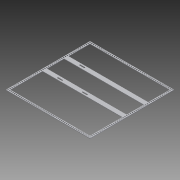
# Autodesk Inventor part: Shooter Mounter
Saved by Autodesk Inventor 2013 (Build 170138000, 138)
## iProperties
Created: 2013-01-17
Part Number: Shooter Mounter
Material: Aluminum 6061
Document SubType Name: Sheet Metal
Designer: actoennies
Mass: 508.006 g
Surface Area: 1380.64 cm^2
Volume: 187.456 cm^3
Density: 2.71 g/cm^3
Sheet Metal Rule: Default
Author: actoennies
Autodesk Inventor part; units mm, degrees
ref_plane "YZ Plane" through (0, 0, 0) normal (1, 0, 0) x (0, 1, 0)
ref_plane "XZ Plane" through (0, 0, 0) normal (0, 1, 0) x (-1, 0, 0)
ref_plane "XY Plane" through (0, 0, 0) normal (0, 0, 1) x (1, 0, 0)
sketch "Sketch1" plane through (0, 0, 0) normal (0, 1, 0) x (-1, 0, 0)
  circle A0 centre (-19.05, -387.35) radius 3.3782
  circle A1 centre (-38.1, -387.35) radius 3.3782
  circle A2 centre (-57.15, -387.35) radius 3.3782
  circle A3 centre (-76.2, -387.35) radius 3.3782
  circle A4 centre (387.35, 11.9063) radius 3.3782
  circle A5 centre (387.35, 35.7188) radius 3.3782
  circle A6 centre (387.35, 59.5313) radius 3.3782
  circle A7 centre (387.35, 83.3438) radius 3.3782
  circle A8 centre (387.35, 0) radius 3.3782
  circle A9 centre (0, -387.35) radius 3.3782
  circle A10 centre (387.35, 95.25) radius 3.3782
  circle A11 centre (387.35, 71.4375) radius 3.3782
  circle A12 centre (387.35, 47.625) radius 3.3782
  circle A13 centre (387.35, 23.8125) radius 3.3782
  circle A14 centre (-85.725, -387.35) radius 3.3782
  circle A15 centre (-66.675, -387.35) radius 3.3782
  circle A16 centre (-47.625, -387.35) radius 3.3782
  circle A17 centre (-28.575, -387.35) radius 3.3782
  circle A18 centre (-9.525, -387.35) radius 3.3782
  line L0 (393.7, 0) -> (393.7, 101.6)
  line L1 (393.7, 101.6) -> (381, 101.6)
  line L2 (0, -381) -> (-88.9, -381)
  line L3 (-101.6, -381) -> (-101.6, -393.7)
  line L4 (-101.6, -393.7) -> (0, -393.7)
  line L5 (-101.6, -393.7) -> (-101.6, 101.6)
  line L6 (-101.6, 101.6) -> (393.7, 101.6)
  line L7 (393.7, 101.6) -> (393.7, -393.7)
  line L8 (393.7, -393.7) -> (-101.6, -393.7)
  line L9 (381, 88.9) -> (381, -381)
  line L10 (381, -381) -> (-88.9, -381)
  line L11 (-88.9, 88.9) -> (381, 88.9)
  line L12 (-88.9, -381) -> (-88.9, 88.9)
  circle A19 centre (387.35, -11.0671) radius 3.3782
  circle A20 centre (387.35, -22.1343) radius 3.3782
  circle A21 centre (387.35, -33.2014) radius 3.3782
  circle A22 centre (387.35, -44.2686) radius 3.3782
  circle A23 centre (387.35, -55.3357) radius 3.3782
  circle A24 centre (387.35, -66.4029) radius 3.3782
  circle A25 centre (387.35, -77.47) radius 3.3782
  circle A26 centre (387.35, -88.5371) radius 3.3782
  circle A27 centre (387.35, -99.6043) radius 3.3782
  circle A28 centre (387.35, -110.6714) radius 3.3782
  circle A29 centre (387.35, -121.7386) radius 3.3782
  circle A30 centre (387.35, -132.8057) radius 3.3782
  circle A31 centre (387.35, -143.8729) radius 3.3782
  circle A32 centre (387.35, -154.94) radius 3.3782
  circle A33 centre (387.35, -166.0071) radius 3.3782
  circle A34 centre (387.35, -177.0743) radius 3.3782
  circle A35 centre (387.35, -188.1414) radius 3.3782
  circle A36 centre (387.35, -199.2086) radius 3.3782
  circle A37 centre (387.35, -210.2757) radius 3.3782
  circle A38 centre (387.35, -221.3429) radius 3.3782
  circle A39 centre (387.35, -232.41) radius 3.3782
  circle A40 centre (387.35, -243.4771) radius 3.3782
  circle A41 centre (387.35, -254.5443) radius 3.3782
  circle A42 centre (387.35, -265.6114) radius 3.3782
  circle A43 centre (387.35, -276.6786) radius 3.3782
  circle A44 centre (387.35, -287.7457) radius 3.3782
  circle A45 centre (387.35, -298.8129) radius 3.3782
  circle A46 centre (387.35, -309.88) radius 3.3782
  circle A47 centre (387.35, -320.9471) radius 3.3782
  circle A48 centre (387.35, -332.0143) radius 3.3782
  circle A49 centre (387.35, -343.0814) radius 3.3782
  circle A50 centre (387.35, -354.1486) radius 3.3782
  circle A51 centre (387.35, -365.2157) radius 3.3782
  circle A52 centre (387.35, -376.2829) radius 3.3782
  circle A53 centre (387.35, -387.35) radius 3.3782
  circle A54 centre (376.2829, -387.35) radius 3.3782
  circle A55 centre (365.2157, -387.35) radius 3.3782
  circle A56 centre (354.1486, -387.35) radius 3.3782
  circle A57 centre (343.0814, -387.35) radius 3.3782
  circle A58 centre (332.0143, -387.35) radius 3.3782
  circle A59 centre (320.9471, -387.35) radius 3.3782
  circle A60 centre (309.88, -387.35) radius 3.3782
  circle A61 centre (298.8129, -387.35) radius 3.3782
  circle A62 centre (287.7457, -387.35) radius 3.3782
  circle A63 centre (276.6786, -387.35) radius 3.3782
  circle A64 centre (265.6114, -387.35) radius 3.3782
  circle A65 centre (254.5443, -387.35) radius 3.3782
  circle A66 centre (243.4771, -387.35) radius 3.3782
  circle A67 centre (232.41, -387.35) radius 3.3782
  circle A68 centre (221.3429, -387.35) radius 3.3782
  circle A69 centre (210.2757, -387.35) radius 3.3782
  circle A70 centre (199.2086, -387.35) radius 3.3782
  circle A71 centre (188.1414, -387.35) radius 3.3782
  circle A72 centre (177.0743, -387.35) radius 3.3782
  circle A73 centre (166.0071, -387.35) radius 3.3782
  circle A74 centre (154.94, -387.35) radius 3.3782
  circle A75 centre (143.8729, -387.35) radius 3.3782
  circle A76 centre (132.8057, -387.35) radius 3.3782
  circle A77 centre (121.7386, -387.35) radius 3.3782
  circle A78 centre (110.6714, -387.35) radius 3.3782
  circle A79 centre (99.6043, -387.35) radius 3.3782
  circle A80 centre (88.5371, -387.35) radius 3.3782
  circle A81 centre (77.47, -387.35) radius 3.3782
  circle A82 centre (66.4029, -387.35) radius 3.3782
  circle A83 centre (55.3357, -387.35) radius 3.3782
  circle A84 centre (44.2686, -387.35) radius 3.3782
  circle A85 centre (33.2014, -387.35) radius 3.3782
  circle A86 centre (22.1343, -387.35) radius 3.3782
  circle A87 centre (11.0671, -387.35) radius 3.3782
  circle A88 centre (377.501, 95.25) radius 3.3782
  circle A89 centre (367.652, 95.25) radius 3.3782
  circle A90 centre (357.8031, 95.25) radius 3.3782
  circle A91 centre (347.9541, 95.25) radius 3.3782
  circle A92 centre (338.1051, 95.25) radius 3.3782
  circle A93 centre (328.2561, 95.25) radius 3.3782
  circle A94 centre (318.4071, 95.25) radius 3.3782
  circle A95 centre (308.5582, 95.25) radius 3.3782
  circle A96 centre (298.7092, 95.25) radius 3.3782
  circle A97 centre (288.8602, 95.25) radius 3.3782
  circle A98 centre (279.0112, 95.25) radius 3.3782
  circle A99 centre (269.1622, 95.25) radius 3.3782
  circle A100 centre (259.3133, 95.25) radius 3.3782
  circle A101 centre (249.4643, 95.25) radius 3.3782
  circle A102 centre (239.6153, 95.25) radius 3.3782
  circle A103 centre (229.7663, 95.25) radius 3.3782
  circle A104 centre (219.9173, 95.25) radius 3.3782
  circle A105 centre (210.0684, 95.25) radius 3.3782
  circle A106 centre (200.2194, 95.25) radius 3.3782
  circle A107 centre (190.3704, 95.25) radius 3.3782
  circle A108 centre (180.5214, 95.25) radius 3.3782
  circle A109 centre (170.6724, 95.25) radius 3.3782
  circle A110 centre (160.8235, 95.25) radius 3.3782
  circle A111 centre (150.9745, 95.25) radius 3.3782
  circle A112 centre (141.1255, 95.25) radius 3.3782
  circle A113 centre (131.2765, 95.25) radius 3.3782
  circle A114 centre (121.4276, 95.25) radius 3.3782
  circle A115 centre (111.5786, 95.25) radius 3.3782
  circle A116 centre (101.7296, 95.25) radius 3.3782
  circle A117 centre (91.8806, 95.25) radius 3.3782
  circle A118 centre (82.0316, 95.25) radius 3.3782
  circle A119 centre (72.1827, 95.25) radius 3.3782
  circle A120 centre (62.3337, 95.25) radius 3.3782
  circle A121 centre (52.4847, 95.25) radius 3.3782
  circle A122 centre (42.6357, 95.25) radius 3.3782
  circle A123 centre (32.7867, 95.25) radius 3.3782
  circle A124 centre (22.9378, 95.25) radius 3.3782
  circle A125 centre (13.0888, 95.25) radius 3.3782
  circle A126 centre (3.2398, 95.25) radius 3.3782
  circle A127 centre (-6.6092, 95.25) radius 3.3782
  circle A128 centre (-16.4582, 95.25) radius 3.3782
  circle A129 centre (-26.3071, 95.25) radius 3.3782
  circle A130 centre (-36.1561, 95.25) radius 3.3782
  circle A131 centre (-46.0051, 95.25) radius 3.3782
  circle A132 centre (-55.8541, 95.25) radius 3.3782
  circle A133 centre (-65.7031, 95.25) radius 3.3782
  circle A134 centre (-75.552, 95.25) radius 3.3782
  circle A135 centre (-85.401, 95.25) radius 3.3782
  circle A136 centre (-95.25, 95.25) radius 3.3782
  circle A137 centre (-95.25, -387.35) radius 3.3782
  circle A138 centre (-95.25, -376.2829) radius 3.3782
  circle A139 centre (-95.25, -365.2157) radius 3.3782
  circle A140 centre (-95.25, -354.1486) radius 3.3782
  circle A141 centre (-95.25, -343.0814) radius 3.3782
  circle A142 centre (-95.25, -332.0143) radius 3.3782
  circle A143 centre (-95.25, -320.9471) radius 3.3782
  circle A144 centre (-95.25, -309.88) radius 3.3782
  circle A145 centre (-95.25, -298.8129) radius 3.3782
  circle A146 centre (-95.25, -287.7457) radius 3.3782
  circle A147 centre (-95.25, -276.6786) radius 3.3782
  circle A148 centre (-95.25, -265.6114) radius 3.3782
  circle A149 centre (-95.25, -254.5443) radius 3.3782
  circle A150 centre (-95.25, -243.4771) radius 3.3782
  circle A151 centre (-95.25, -232.41) radius 3.3782
  circle A152 centre (-95.25, -221.3429) radius 3.3782
  circle A153 centre (-95.25, -210.2757) radius 3.3782
  circle A154 centre (-95.25, -199.2086) radius 3.3782
  circle A155 centre (-95.25, -188.1414) radius 3.3782
  circle A156 centre (-95.25, -177.0743) radius 3.3782
  circle A157 centre (-95.25, -166.0071) radius 3.3782
  circle A158 centre (-95.25, -154.94) radius 3.3782
  circle A159 centre (-95.25, -143.8729) radius 3.3782
  circle A160 centre (-95.25, -132.8057) radius 3.3782
  circle A161 centre (-95.25, -121.7386) radius 3.3782
  circle A162 centre (-95.25, -110.6714) radius 3.3782
  circle A163 centre (-95.25, -99.6043) radius 3.3782
  circle A164 centre (-95.25, -88.5371) radius 3.3782
  circle A165 centre (-95.25, -77.47) radius 3.3782
  circle A166 centre (-95.25, -66.4029) radius 3.3782
  circle A167 centre (-95.25, -55.3357) radius 3.3782
  circle A168 centre (-95.25, -44.2686) radius 3.3782
  circle A169 centre (-95.25, -33.2014) radius 3.3782
  circle A170 centre (-95.25, -22.1343) radius 3.3782
  circle A171 centre (-95.25, -11.0671) radius 3.3782
  circle A172 centre (-95.25, 0) radius 3.3782
  line L13 (146.05, 23.8125) -> (146.05, -246.8553) construction
  circle A173 centre (-95.25, 11.9063) radius 3.3782
  circle A174 centre (-95.25, 23.8125) radius 3.3782
  circle A175 centre (-95.25, 47.625) radius 3.3782
  circle A176 centre (-95.25, 59.5313) radius 3.3782
  circle A177 centre (-95.25, 71.4375) radius 3.3782
  circle A178 centre (-95.25, 83.3438) radius 3.3782
  circle A179 centre (-95.25, 35.7188) radius 3.3782
  point P0 (0, 0)
  dimension "d0" = 12.7
  dimension "d3" = 12.7
  dimension "d4" = 12.7
  dimension "d6" = 393.7
  dimension "d9" = 11.0671
  dimension "d16" = 11.0671
  dimension "d21" = 488.95
  dimension "d24" = 9.849
  dimension "d36" = 393.7
  dimension "d42" = 11.0671
  dimension "d43" = 6.35
  dimension "d46" = 11.0671
  dimension "d51" = 469.9
  dimension "d52" = 234.95
  constraints: 180 centre point, 28 end point, 7 symmetric about line, 6 horizontal, 4 vertical, 3 perpendicular, 2 collinear, 1 parallel, 313 other
  measures "d0" distance between parallel lines of L6 L11
  measures "d3" distance between parallel lines of L9 L7
  measures "d4" distance between parallel lines of L8 L10
  measures "d6" distance from line of L8 A8.centre
  measures "d9" distance of A8.centre A19.centre
  measures "d16" distance of A53.centre A54.centre
  measures "d21" distance from line of A10.centre L5
  measures "d24" distance of A10.centre A88.centre
  measures "d36" distance from line of L7 A9.centre
  measures "d42" distance of A52.centre A53.centre
  measures "d43" distance from line of L6 A136.centre
  measures "d46" distance of A137.centre A138.centre
  measures "d51" distance between parallel lines of L9 L12
  measures "d52" distance between parallel lines of L9 L13
extrude "Extrusion2" add sketch "Sketch1" along normal blind 3.175
sketch "Sketch2" plane through (0, 3.175, 0) normal (0, 1, 0) x (1, 0, 0)
  line L0 (-381, 381) -> (88.9, 381)
  line L1 (88.9, 381) -> (88.9, -88.9)
  line L2 (-381, -88.9) -> (-381, 381)
  line L3 (-381, 254) -> (88.9, 254)
  line L4 (-381, 228.6) -> (88.9, 228.6)
  line L5 (-381, 127) -> (88.9, 127)
  line L6 (-381, 101.6) -> (88.9, 101.6)
  point P0 (0, 0)
  dimension "d55" = 25.4
  dimension "d58" = 25.4
  dimension "d59" = 127
  dimension "d60" = 101.6
  measures "d55" distance between parallel lines of L3 L4
  measures "d58" distance between parallel lines of L6 L5
  measures "d59" distance between parallel lines of L0 L3
  measures "d60" distance between parallel lines of L4 L5
sheet face with bend "Face1" sketch "Sketch2" thickness 3.175 toward (0, -1, 0) bend radius 3.175 relief tear relief width 3.175 relief depth 1.5875 contours L3 L1 L4 L2 | L5 L1 L6 L2
bend "Bend1"
sketch "Sketch3" plane through (0, 0, 0) normal (0, -1, 0) x (1, 0, 0)
  ellipse E0 centre (-142.5318, -113.9531) end of major axis (-145.91, -113.9531) minor radius 3.2325 projected
  point P0 (0, 0)
  constraints: 1 other
extrude "Cut1" cut sketch "Sketch3" against normal blind 3.175
sketch "Sketch4" plane through (0, 3.175, 0) normal (0, 1, 0) x (1, 0, 0)
  ellipse E0 centre (-288.3202, 113.4978) end of major axis (-291.6984, 113.4978) minor radius 3.2325 projected
  ellipse E1 centre (-288.3202, 238.0592) end of major axis (-291.6984, 238.0592) minor radius 3.2325 projected
  point P0 (0, 0)
  constraints: 2 other
extrude "Cut2" cut sketch "Sketch4" against normal blind 3.175
sketch "Sketch5" plane through (0, 3.175, 0) normal (0, 1, 0) x (1, 0, 0)
  circle A0 centre (-288.3202, 242.57) radius 3.3782 projected
  circle A1 centre (-288.3202, 112.395) radius 3.3782 projected
  circle A2 centre (-142.5318, 112.395) radius 3.3782 projected
  line L0 (-381, 101.6) -> (88.9, 101.6) projected
  line L1 (88.9, 254) -> (-381, 254) projected
  arc A3 (-155.2318, 115.7732) -> (-155.2318, 109.0168) centre (-155.2318, 112.395) ccw
  arc A4 (-129.8318, 109.0168) -> (-129.8318, 115.7732) centre (-129.8318, 112.395) ccw
  arc A5 (-301.0202, 115.7732) -> (-301.0202, 109.0168) centre (-301.0202, 112.395) ccw
  arc A6 (-275.6202, 109.0168) -> (-275.6202, 115.7732) centre (-275.6202, 112.395) ccw
  arc A7 (-301.0202, 245.9542) -> (-301.0202, 239.1858) centre (-301.0202, 242.57) ccw
  arc A8 (-275.6202, 239.1858) -> (-275.6202, 245.9542) centre (-275.6202, 242.57) ccw
  line L2 (-301.0202, 245.9542) -> (-275.6202, 245.9542)
  line L3 (-301.0202, 239.1858) -> (-275.6202, 239.1858)
  line L4 (-301.0202, 115.7732) -> (-275.6202, 115.7732)
  line L5 (-275.6202, 109.0168) -> (-301.0202, 109.0168)
  line L6 (-155.2318, 115.7732) -> (-129.8318, 115.7732)
  line L7 (-129.8318, 109.0168) -> (-155.2318, 109.0168)
  point P0 (0, 0)
  dimension "d70" = 6.7564
  dimension "d71" = 6.7564
  dimension "d72" = 12.7
  dimension "d73" = 12.7
  dimension "d74" = 10.795
  dimension "d75" = 10.795
  dimension "d76" = 10.795
  dimension "d77" = 10.795
  dimension "d78" = 10.795
  dimension "d79" = 12.7
  dimension "d80" = 12.7
  dimension "d81" = 6.7564
  dimension "d82" = 6.7564
  dimension "d83" = 11.43
  dimension "d84" = 11.43
  dimension "d85" = 11.43
  dimension "d86" = 12.7
  dimension "d87" = 12.7
  dimension "d88" = 6.7684
  dimension "d89" = 6.7684
  constraints: 12 end point, 12 point on circle, 7 tangent, 6 centre point, 2 parallel
  measures "d70" diameter of A5
  measures "d71" diameter of A6
  measures "d72" distance of A6.centre A1.centre
  measures "d73" distance of A1.centre A5.centre
  measures "d74" distance from line of L0 A1.centre
  measures "d75" distance from line of L0 A5.centre
  measures "d76" distance from line of L0 A6.centre
  measures "d77" distance from line of L0 A4.centre
  measures "d78" distance from line of L0 A3.centre
  measures "d79" distance of A4.centre A2.centre
  measures "d80" distance of A2.centre A3.centre
  measures "d81" diameter of A3
  measures "d82" diameter of A4
  measures "d83" distance from line of L1 A0.centre
  measures "d84" distance from line of L1 A7.centre
  measures "d85" distance from line of L1 A8.centre
  measures "d86" distance of A8.centre A0.centre
  measures "d87" distance of A7.centre A0.centre
  measures "d88" diameter of A7
  measures "d89" diameter of A8
extrude "Cut3" cut sketch "Sketch5" against normal blind 3.175 contours A1 L4 A6 L5 | A1 L5 A5 L4 | A2 L6 A4 L7 | A2 L7 A3 L6 | L2 A8 L3 A7
equation "\"d46\" = d42"
equation "\"d52\" = 0.5 * d51"
equation "\"d66\" = Thickness"
equation "\"d68\" = Thickness"
equation "\"d75\" = d74"
equation "\"d76\" = d74"
equation "\"d77\" = d74"
equation "\"d78\" = d74"
equation "\"d84\" = d83"
equation "\"d85\" = d83"
equation "\"d90\" = Thickness"
equation "\"d61\" = BendRadius"
equation "\"d62\" = BendReliefWidth"
equation "\"d64\" = MinimumRemnant"
equation "\"d63\" = BendReliefDepth"
equation "\"d65\" = BendRadius"
equation "\"BendRadius\" = Thickness"
equation "\"BendReliefWidth\" = Thickness"
equation "\"BendReliefDepth\" = 0.5 * Thickness"
equation "\"CornerReliefSize\" = 4 * Thickness"
equation "\"MinimumRemnant\" = 2 * Thickness"
equation "\"TransitionRadius\" = BendRadius"
equation "\"JacobiRadiusSize\" = Thickness"
equation "\"GapSize\" = Thickness"
equation "\"Thickness\" = 3.175"
body "Solid2"
